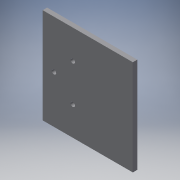
# Autodesk Inventor part: Pan cross bar spacer
Saved by Autodesk Inventor 2018 (Build 220112000, 112)
## iProperties
Created: 2018-06-26
Part Number: Pan cross bar spacer
Material: Generic
Document SubType Name: Modeling
Designer: Ajith Thomas
Density: 1 g/cm^3
Appearance: Default
Author: Ajith Thomas
Autodesk Inventor part; units mm, degrees
ref_plane "YZ Plane" through (0, 0, 0) normal (1, 0, 0) x (0, 1, 0)
ref_plane "XZ Plane" through (0, 0, 0) normal (0, 1, 0) x (-1, 0, 0)
ref_plane "XY Plane" through (0, 0, 0) normal (0, 0, 1) x (1, 0, 0)
sketch "Sketch1" plane through (0, 0, 0) normal (0, 0, 1) x (1, 0, 0)
  line L0 (0, 0) -> (0, 63.5) construction
  line L1 (60, 0) -> (60, 63.5) construction
  line L2 (18, 66.5) -> (42, 66.5) construction
  line L3 (42, 0) -> (18, 0) construction
  circle A0 centre (20, 19.25) radius 1.5 projected
  circle A1 centre (10.45, 31.75) radius 1.35 construction
  circle A2 centre (20, 44.25) radius 1.5 projected
  line L4 (0, 0) -> (60, 0)
  line L5 (60, 0) -> (60, 63.5)
  line L6 (60, 63.5) -> (0, 63.5)
  line L7 (0, 63.5) -> (0, 0)
  circle A3 centre (20, 44.25) radius 1.5 projected
  circle A4 centre (7.5, 31.75) radius 1.5 projected
  circle A5 centre (20, 19.25) radius 1.5 projected
  line L8 (60, 0) -> (42, 0) projected
  line L9 (60, 0) -> (60, 63.5) projected
  line L10 (42, 63.5) -> (60, 63.5) projected
  line L11 (42, 63.5) -> (42, 66.5) projected
  line L12 (18, 66.5) -> (42, 66.5) projected
  line L13 (18, 63.5) -> (18, 66.5) projected
  line L14 (0, 63.5) -> (18, 63.5) projected
  line L15 (0, 0) -> (0, 63.5) projected
  line L16 (18, 0) -> (0, 0) projected
  line L17 (18, 0) -> (18, -3) projected
  line L18 (18, -3) -> (42, -3) projected
  line L19 (42, 0) -> (42, -3) projected
  constraints: 8 end point, 2 parallel, 1 horizontal, 1 perpendicular
extrude "Extrusion2" add sketch "Sketch1" along normal blind 3 contours L7 L6 L5 L4
body "Solid2"
